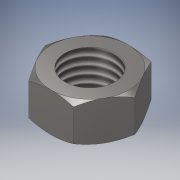
# Autodesk Inventor part: Hinge Pin Nut
Saved by Autodesk Inventor 2018 (Build 220112000, 112)
## iProperties
Created: 2016-10-27
Part Number: Hinge Pin Nut
Material: Steel, Carbon
Document SubType Name: Modeling
Designer: Joey
Density: 7.85 g/cm^3
Appearance: Semi-Polished
Mass: 166.052 g
Surface Area: 67.5398 cm^2
Volume: 21.1531 cm^3
Author: Joey
Autodesk Inventor part; units mm, degrees
ref_plane "YZ Plane" through (0, 0, 0) normal (1, 0, 0) x (0, 1, 0)
ref_plane "XZ Plane" through (0, 0, 0) normal (0, 1, 0) x (-1, 0, 0)
ref_plane "XY Plane" through (0, 0, 0) normal (0, 0, 1) x (1, 0, 0)
sketch "Sketch3" plane through (0, 0, 0) normal (0, 1, 0) x (-1, 0, 0)
  line L0 (14.6647, 0) -> (7.3323, -12.7)
  line L1 (7.3323, -12.7) -> (-7.3323, -12.7)
  line L2 (-7.3323, -12.7) -> (-14.6647, 0)
  line L3 (-14.6647, 0) -> (-7.3323, 12.7)
  line L4 (-7.3323, 12.7) -> (7.3323, 12.7)
  line L5 (7.3323, 12.7) -> (14.6647, 0)
  point P0 (0, 0)
  point P1 (0, 0)
  point P2 (0, 0)
  dimension "d27" = 25.4
  constraints: 12 end point, 2 coincident, 1 horizontal, 13 other
  measures "d27" distance between parallel lines of L4 L1
extrude "Extrusion2" add sketch "Sketch3" along normal mid plane 12.7
sketch "Sketch5" plane through (0, 0, 0) normal (0, 0, 1) x (1, 0, 0)
  line L0 (0, -17.78) -> (0, 17.78) projected
  line L1 (14.6647, 6.35) -> (7.3323, 6.35) construction
  line L2 (7.3323, 6.35) -> (7.3323, -6.35) projected
  line L3 (14.6647, 6.35) -> (7.3323, 6.35) projected
  line L4 (14.6647, 6.35) -> (14.6647, -6.35) construction
  line L5 (7.3323, -6.35) -> (14.6647, -6.35) projected
  line L6 (12.7, 6.35) -> (14.6647, 6.35)
  line L7 (14.6647, 6.35) -> (14.6647, 5.2157)
  line L8 (14.6647, 5.2157) -> (12.7, 6.35)
  line L9 (0, 0) -> (14.3088, 0) construction
  line L10 (12.7, -6.35) -> (14.6647, -6.35)
  line L11 (14.6647, -6.35) -> (14.6647, -5.2157)
  line L12 (14.6647, -5.2157) -> (12.7, -6.35)
  dimension "d15" = 25.4
  dimension "d16" = 30
  constraints: 14 end point, 3 symmetric about line, 2 collinear, 2 horizontal, 1 perpendicular
  measures "d15" diameter of L6.start L0
  measures "d16" angle of L8 L6
revolve "Revolution3" cut sketch "Sketch5" angle 360 about axis through (0, -10, 0) along (0, 1, 0)
hole "Hole1" at (0, 6.35, 0) direction (0, -1, 0) diameter 16.3068 end through all thread size "3/4-10 UNC" class "2B" standard "ANSI Unified Screw Threads"
equation "\"diameter\" = 25.4"
equation "\"length\" = 76.2"
body "Solid1"
